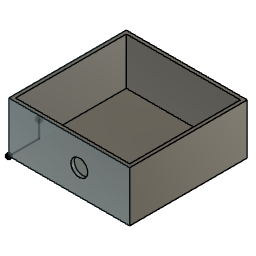
ecg 1 v1 (Autodesk Fusion 360 design; units mm, degrees)
Autodesk Fusion 360 part; units mm, degrees
sketch "Sketch1" plane through (0, 0, 0) normal (0, 0, 1) x (1, 0, 0)
  line L0 (36, 35) -> (-36, 35)
  line L1 (-36, 35) -> (-36, -35)
  line L2 (-36, -35) -> (36, -35)
  line L3 (36, -35) -> (36, 35)
  line L4 (36, 35) -> (-36, -35) construction
  line L5 (-36, 35) -> (36, -35) construction
  dimension "d1" = 72
  dimension "d2" = 70
  constraint horizontal L0
  constraint perpendicular L0 L1
  constraint parallel L0 L2
  constraint parallel L1 L3
  constraint coincident L4 origin
  constraint coincident L5 origin
  measures "d1" distance of L1.end L2.end
  measures "d2" distance of L0.end L1.end
extrude "Extrude1" add sketch "Sketch1" along normal blind 30
shell "Shell1" thickness 2 removed faces 1 at (-12, 11.6667, 30)
sketch "Sketch2" plane through (-36, 0, 0) normal (-1, 0, 0) x (0, -1, 0)
  line L0 (-35, 0) -> (35, 0)
  line L1 (35, 0) -> (35, 30)
  line L2 (35, 30) -> (-35, 30)
  line L3 (-35, 30) -> (-35, 0)
  line L4 (35, 0) -> (17, 0)
  line L5 (17, 0) -> (17, 10)
  dimension "d11" = 18
  dimension "d12" = 10
  constraint coincident L0.end L1.start
  constraint perpendicular L1 L4
  constraint perpendicular L4 L5
  measures "d11" distance of L0.end L4.end
  measures "d12" distance of L4.end L5.end
hole "Hole2" at (-36, -17.0122, 10.0373) direction (1, 0, 0) diameter 5 depth 2 tip angle 118
sketch "Sketch3" plane through (0, -35, 0) normal (0, -1, 0) x (1, 0, 0)
  line L0 (-36, 0) -> (36, 0)
  line L1 (36, 0) -> (36, 30)
  line L2 (36, 30) -> (-36, 30)
  line L3 (-36, 30) -> (-36, 0)
hole "Hole3" at (6, -35, 15) direction (0, 1, 0) diameter 10 depth 2 tip angle 118
